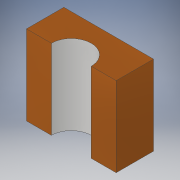
# Autodesk Inventor part: reverse gear lower base bearing holder
Saved by Autodesk Inventor 2017 (Build 210142000, 142)
## iProperties
Created: 2018-10-30
Part Number: reverse gear lower base bearing holder
Material: Generic
Document SubType Name: Modeling
Designer: User
Density: 1 g/cm^3
Appearance: Default
Author: User
Autodesk Inventor part; units mm, degrees
ref_plane "YZ Plane" through (0, 0, 0) normal (1, 0, 0) x (0, 1, 0)
ref_plane "XZ Plane" through (0, 0, 0) normal (0, 1, 0) x (-1, 0, 0)
ref_plane "XY Plane" through (0, 0, 0) normal (0, 0, 1) x (1, 0, 0)
sketch "Sketch1" plane through (0, 0, 0) normal (0, 1, 0) x (-1, 0, 0)
  line L0 (0, 0) -> (0, -16)
  line L1 (0, -16) -> (-18, -16)
  line L2 (-18, -16) -> (-18, 0)
  line L3 (-18, 0) -> (0, 0)
  dimension "d1" = 18
  dimension "d2" = 16
  dimension "d3" = 18
  constraints: 8 end point, 2 perpendicular, 1 horizontal, 1 vertical
  measures "d1" distance of L0.end L1.end
  measures "d2" distance of L1.end L2.end
  measures "d3" distance of L2.end L0.start
extrude "Extrusion1" add sketch "Sketch1" along normal blind 7.5
sketch "Sketch2" plane through (0, 0, 0) normal (0, 0, 1) x (1, 0, 0)
  line L0 (18, 0) -> (0, 0) projected
  line L1 (18, 0) -> (18, 7.5) projected
  line L2 (0, 7.5) -> (18, 7.5) projected
  line L3 (0, 0) -> (0, 7.5) projected
  line L4 (18, 0) -> (0, 0) projected
  line L5 (13, 0) -> (5, 0)
  circle A0 centre (9, 0) radius 4
  dimension "d8" = 8
  constraints: 2 end point, 2 point on line, 1 centre point, 1 collinear, 1 midpoint
  measures "d8" diameter of A0
extrude "Extrusion2" cut sketch "Sketch2" against normal through all contours A0 L0 | L0 A0
body "Solid1"
